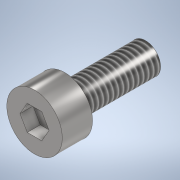
# Autodesk Inventor part: M3-8
Saved by Autodesk Inventor 2022 (Build 260153000, 153)
## iProperties
Part Number: M3-8
Material: ステンレス鋼 AISI 304
Document SubType Name: Modeling
Designer: Masato Kubotera
Density: 6.3912 g/cm^3
Appearance: 半つや出し
Mass: 0.543 g
Surface Area: 1.56805 cm^2
Volume: 0.0849605 cm^3
Description: ReadyMade
Author: Masato Kubotera
Comments: Width across flats : 2.5
Autodesk Inventor part; units mm, degrees
ref_plane "YZ Plane" through (0, 0, 0) normal (1, 0, 0) x (0, 1, 0)
ref_plane "XZ Plane" through (0, 0, 0) normal (0, 1, 0) x (-1, 0, 0)
ref_plane "XY Plane" through (0, 0, 0) normal (0, 0, 1) x (1, 0, 0)
sketch "スケッチ1" plane through (0, 0, 0) normal (1, 0, 0) x (0, 1, 0)
  line L0 (0, 11) -> (0, 0)
  line L1 (0, 0) -> (2.75, 0)
  line L2 (2.75, 0) -> (2.75, 3)
  line L3 (2.75, 3) -> (1.5, 3)
  line L4 (1.5, 3) -> (1.5, 11)
  line L5 (1.5, 11) -> (0, 11)
  dimension "d2" = 3
  dimension "d10" = 8
  dimension "d11" = 3
  dimension "d12" = 5.5
  constraints: 12 end point, 5 perpendicular, 1 vertical
  measures "d2" distance of L1.end L2.end
  measures "d10" distance of L3.end L4.end
  measures "d11" diameter of L4 L0
  measures "d12" diameter of L2 L0
revolve "回転1" add sketch "スケッチ1" angle 360 about axis through (0, 0, 11) along (0, 0, -1)
thread "ねじ1" size "M3x0.5" class "6g" standard "ANSI Metric M Profile" full length
sketch "スケッチ2" plane through (0, 0, 0) normal (0, 0, -1) x (-1, 0, 0)
  line L0 (0, 1.4434) -> (1.25, 0.7217)
  line L1 (1.25, 0.7217) -> (1.25, -0.7217)
  line L2 (1.25, -0.7217) -> (0, -1.4434)
  line L3 (0, -1.4434) -> (-1.25, -0.7217)
  line L4 (-1.25, -0.7217) -> (-1.25, 0.7217)
  line L5 (-1.25, 0.7217) -> (0, 1.4434)
  circle A0 centre (0, 0) radius 2.75 projected
  line L6 (0, 2.75) -> (0, -2.75) construction
  dimension "d7" = 2.5
  constraints: 14 end point, 2 point on circle, 1 coincident, 1 midpoint, 1 point on line, 1 vertical, 13 other
  measures "d7" distance between parallel lines of L1 L4
extrude "押し出し1" cut sketch "スケッチ2" against normal blind 1.3 contours L0 L1 L2 L3 L4 L5
